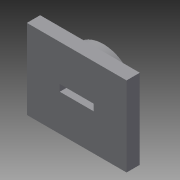
# Autodesk Inventor part: LDR_case
Saved by Autodesk Inventor 2015 SP2 (Build 190223200, 223)
## iProperties
Created: 2016-09-05
Part Number: LDR_case
Material: Generic
Document SubType Name: Modeling
Designer: jm799
Density: 1 g/cm^3
Appearance: Default
Author: jm799
Autodesk Inventor part; units mm, degrees
ref_plane "YZ Plane" through (0, 0, 0) normal (1, 0, 0) x (0, 1, 0)
ref_plane "XZ Plane" through (0, 0, 0) normal (0, 1, 0) x (-1, 0, 0)
ref_plane "XY Plane" through (0, 0, 0) normal (0, 0, 1) x (1, 0, 0)
sketch "Sketch1" plane through (0, 0, 0) normal (0, 1, 0) x (-1, 0, 0)
  line L0 (2.55, 0.5) -> (-2.55, 0.5)
  line L1 (-2.55, 0.5) -> (-2.55, -0.5)
  line L2 (-2.55, -0.5) -> (2.55, -0.5)
  line L3 (2.55, -0.5) -> (2.55, 0.5)
  line L4 (-2.55, 0) -> (2.55, 0) construction
  point P0 (0, 0)
  point P1 (0, -0.5)
  point P2 (0, 0)
  dimension "d0" = 5.1
  dimension "d1" = 1
  constraints: 10 end point, 4 midpoint, 2 parallel, 1 coincident, 1 horizontal, 1 perpendicular
  measures "d0" distance of L2.end L1.end
  measures "d1" distance of L1.end L0.end
sketch "Sketch2" plane through (0, 0, 0) normal (0, 1, 0) x (-1, 0, 0)
  circle A0 centre (0, 0) radius 5
  dimension "d4" = 10
  constraints: 1 centre point, 1 coincident
  measures "d4" diameter of A0
sketch "Sketch3" plane through (0, 0, 0) normal (0, 1, 0) x (-1, 0, 0)
  line L0 (7.5, -6) -> (-7.5, -6)
  line L1 (-7.5, -6) -> (-7.5, 6)
  line L2 (-7.5, 6) -> (7.5, 6)
  line L3 (7.5, 6) -> (7.5, -6)
  line L4 (7.5, 0) -> (-7.5, 0) construction
  line L5 (0, -6) -> (0, 6) construction
  point P0 (0, 0)
  point P1 (0, 0)
  dimension "d2" = 15
  dimension "d3" = 12
  constraints: 12 end point, 5 midpoint, 2 parallel, 1 coincident, 1 horizontal, 1 perpendicular
  measures "d2" distance of L0.start L0.end
  measures "d3" distance of L2.end L0.start
extrude "Extrusion1" add sketch "Sketch3" along normal blind 2
extrude "Extrusion2" cut sketch "Sketch1" along normal blind 2
extrude "Extrusion4" add sketch "Sketch2" along normal blind 4
sketch "Sketch7" plane through (0, 4, 0) normal (0, 1, 0) x (1, 0, 0)
  circle A0 centre (0, 0) radius 4.4878
  constraints: 1 centre point, 1 coincident
extrude "Extrusion5" cut sketch "Sketch7" against normal blind 3
sketch "Sketch8" plane through (0, 1, 0) normal (0, 1, 0) x (1, 0, 0)
  line L0 (-2.55, 0.5) -> (2.55, 0.5)
  line L1 (2.55, 0.5) -> (2.55, -0.5)
  line L2 (2.55, -0.5) -> (-2.55, -0.5)
  line L3 (-2.55, -0.5) -> (-2.55, 0.5)
  line L4 (-2.55, 0) -> (2.55, 0) construction
  line L5 (0, 0.5) -> (0, -0.5) construction
  point P0 (0, 0)
  point P1 (0, 0)
  dimension "d15" = 5.1
  dimension "d16" = 1
  constraints: 12 end point, 5 midpoint, 2 parallel, 1 coincident, 1 horizontal, 1 perpendicular
  measures "d15" distance of L1.end L2.end
  measures "d16" distance of L0.end L1.end
extrude "Extrusion6" cut sketch "Sketch8" against normal blind 3
body "Solid1"
